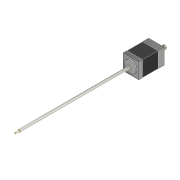
# Autodesk Inventor part: maly_silnik
Saved by Autodesk Inventor 2021 (Build 250183000, 183)
## iProperties
Created: 2022-05-17
Part Number: maly_silnik
Material: Generic
Document SubType Name: Modeling
Designer: agnpi
Density: 1 g/cm^3
Appearance: Default
Author: agnpi
Autodesk Inventor part; units mm, degrees
ref_plane "YZ Plane" through (0, 0, 0) normal (1, 0, 0) x (0, 1, 0)
ref_plane "XZ Plane" through (0, 0, 0) normal (0, 1, 0) x (-1, 0, 0)
ref_plane "XY Plane" through (0, 0, 0) normal (0, 0, 1) x (1, 0, 0)
sketch "Sketch1" plane through (0, 0, 0) normal (0, 0, 1) x (1, 0, 0)
  line L0 (-14.14, 0) -> (14.14, 0) projected
  line L1 (0, -14.14) -> (0, 14.14) projected
  line L2 (10.1, 10.1) -> (-10.1, 10.1)
  line L3 (-10.1, 10.1) -> (-10.1, -10.1)
  line L4 (-10.1, -10.1) -> (10.1, -10.1)
  line L5 (10.1, -10.1) -> (10.1, 10.1)
  line L6 (10.1, 10.1) -> (-10.1, -10.1) construction
  line L7 (-10.1, 10.1) -> (10.1, -10.1) construction
  point P0 (0, 0)
  dimension "d0" = 20.2
  dimension "d1" = 20.2
  constraints: 12 end point, 2 midpoint, 2 parallel, 1 horizontal, 1 perpendicular
  measures "d0" distance of L4.end L3.end
  measures "d1" distance between parallel lines of L2 L4
extrude "Extrusion3" add sketch "Sketch1" along normal blind 8
sketch "Sketch3" plane through (0, 0, 8) normal (0, 0, 1) x (1, 0, 0)
  line L0 (-10.1, -10.1) -> (10.1, -10.1) projected
  line L1 (-10.1, 10.1) -> (10.1, 10.1)
  line L2 (10.1, 10.1) -> (10.1, -10.1)
  line L3 (10.1, -10.1) -> (-10.1, -10.1)
  line L4 (-10.1, -10.1) -> (-10.1, 10.1)
  line L5 (-10.1, 10.1) -> (10.1, -10.1) construction
  line L6 (10.1, 10.1) -> (-10.1, -10.1) construction
  point P0 (0, 0)
  constraints: 12 end point, 2 midpoint, 2 parallel, 1 horizontal, 1 perpendicular
extrude "Extrusion4" add sketch "Sketch3" along normal blind 20 separate body
sketch "Sketch4" plane through (0, 0, 28) normal (0, 0, 1) x (1, 0, 0)
  line L0 (-10.1, -10.1) -> (10.1, -10.1) projected
  line L1 (-10.1, 10.1) -> (10.1, 10.1)
  line L2 (10.1, 10.1) -> (10.1, -10.1)
  line L3 (10.1, -10.1) -> (-10.1, -10.1)
  line L4 (-10.1, -10.1) -> (-10.1, 10.1)
  line L5 (-10.1, 10.1) -> (10.1, -10.1) construction
  line L6 (10.1, 10.1) -> (-10.1, -10.1) construction
  point P0 (0, 0)
  constraints: 12 end point, 2 midpoint, 2 parallel, 1 horizontal, 1 perpendicular
extrude "Extrusion5" add sketch "Sketch4" along normal blind 5 separate body
sketch "Sketch5" plane through (0, 0, 33) normal (0, 0, 1) x (1, 0, 0)
  circle A0 centre (0, 0) radius 7.5
  dimension "d12" = 15
  constraints: 1 centre point, 1 coincident
  measures "d12" diameter of A0
extrude "Extrusion6" add sketch "Sketch5" along normal blind 1.5 separate body
sketch "Sketch6" plane through (0, 0, 0) normal (0, 0, -1) x (-1, 0, 0)
  circle A0 centre (0, 0) radius 2.5
  dimension "d15" = 5
  constraints: 1 centre point, 1 coincident
  measures "d15" diameter of A0
extrude "Extrusion7" add sketch "Sketch6" along normal blind 10.7 separate body
sketch "Sketch7" plane through (0, 0, 34.5) normal (0, 0, 1) x (1, 0, 0)
  circle A0 centre (0, 0) radius 1.75
  dimension "d18" = 3.5
  constraints: 1 centre point, 1 coincident
  measures "d18" diameter of A0
extrude "Extrusion8" add sketch "Sketch7" along normal blind 143.5 separate body
sketch "Sketch8" plane through (0, 0, 178) normal (0, 0, 1) x (1, 0, 0)
  circle A0 centre (0, 0) radius 1
  dimension "d21" = 2
  constraints: 1 centre point, 1 coincident
  measures "d21" diameter of A0
extrude "Extrusion9" add sketch "Sketch8" along normal blind 5 bodies 6
body "Solid2"
body "Solid3"
body "Solid4"
body "Solid5"
body "Solid6"
body "Solid7"
